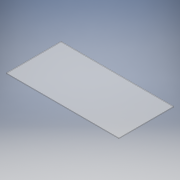
# Autodesk Inventor part: 左右
Saved by Autodesk Inventor 2018 (Build 220112000, 112)
## iProperties
Created: 2017-10-08
Part Number: 左右
Material: 一般
Document SubType Name: Modeling
Designer: mura5
Density: 1 g/cm^3
Appearance: ポリカーボネート - クリア
Author: mura5
Autodesk Inventor part; units mm, degrees
ref_plane "YZ Plane" through (0, 0, 0) normal (1, 0, 0) x (0, 1, 0)
ref_plane "XZ Plane" through (0, 0, 0) normal (0, 1, 0) x (-1, 0, 0)
ref_plane "XY Plane" through (0, 0, 0) normal (0, 0, 1) x (1, 0, 0)
sketch "スケッチ1" plane through (0, 0, 0) normal (0, 0, 1) x (1, 0, 0)
  line L0 (-308.5333, -150) -> (308.5333, -150)
  line L1 (308.5333, -150) -> (308.5333, 150)
  line L2 (308.5333, 150) -> (-308.5333, 150)
  line L3 (-308.5333, 150) -> (-308.5333, -150)
  line L4 (-308.5333, -150) -> (308.5333, 150) construction
  line L5 (308.5333, -150) -> (-308.5333, 150) construction
  point P0 (0, 0)
  dimension "d0" = 617.0667
  dimension "d1" = 300
  constraints: 12 end point, 2 midpoint, 2 parallel, 1 horizontal, 1 perpendicular
  measures "d0" distance of L1.end L2.end
  measures "d1" distance of L0.end L1.end
extrude "押し出し1" add sketch "スケッチ1" along normal blind 4
